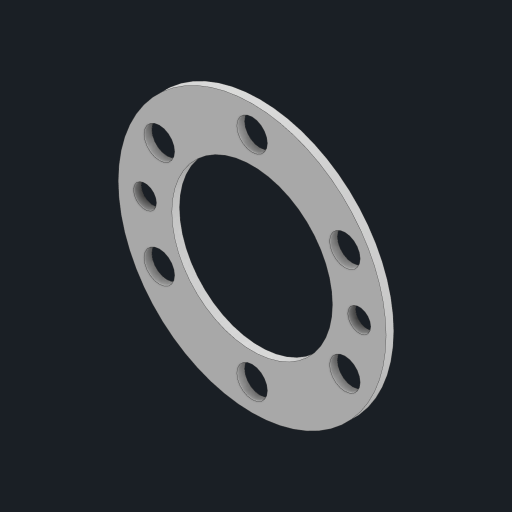
# Autodesk Inventor part: AK80Head
Saved by Autodesk Inventor 2023 (Build 270158000, 158)
## iProperties
Created: 2023-03-31
Part Number: AK80Head
Material: Generic
Document SubType Name: Modeling
Designer: valer
Density: 1 g/cm^3
Appearance: Default
Author: valer
Autodesk Inventor part; units mm, degrees
ref_plane "YZ Plane" through (0, 0, 0) normal (1, 0, 0) x (0, 1, 0)
ref_plane "XZ Plane" through (0, 0, 0) normal (0, 1, 0) x (-1, 0, 0)
sketch "Sketch1" plane through (0, 0, 0) normal (0, 0, 1) x (1, 0, 0)
  circle A0 centre (0, 0) radius 49
  circle A1 centre (0, 0) radius 44.5
  circle A2 centre (0, 0) radius 14 construction
  line L0 (0, 0) -> (0, 49.9271) construction
  line L1 (0, 0) -> (49, 0) construction
  line L2 (0, 0) -> (-49, 0) construction
  circle A3 centre (14, 0) radius 1.5
  circle A4 centre (-14, 0) radius 1.5
  circle A5 centre (0, 14) radius 2
  circle A6 centre (0, 44.5) radius 1.5
  circle A7 centre (44.5, 0) radius 1.5
  circle A8 centre (-44.5, 0) radius 1.5
  line L3 (0, 0) -> (-12.1244, 7) construction
  circle A9 centre (-12.1244, 7) radius 2
  circle A10 centre (12.1244, 7) radius 2
  circle A11 centre (0, -14) radius 2
  circle A12 centre (-12.1244, -7) radius 2
  circle A13 centre (12.1244, -7) radius 2
  line L4 (0, 0) -> (-31.4663, 31.4663) construction
  circle A14 centre (-31.4663, 31.4663) radius 1.5
  circle A15 centre (31.4663, 31.4663) radius 1.5
  circle A16 centre (0, -44.5) radius 1.5
  circle A17 centre (-31.4663, -31.4663) radius 1.5
  circle A18 centre (31.4663, -31.4663) radius 1.5
  circle A19 centre (0, 0) radius 10.5
  circle A20 centre (0, 0) radius 17.5
  circle A21 centre (0, 0) radius 36
  circle A22 centre (0, 0) radius 40
  circle A23 centre (0, 0) radius 5
  dimension "d0" = 98
  dimension "d1" = 89
  dimension "d2" = 28
  dimension "d3" = 3
  dimension "d4" = 3
  dimension "d5" = 4
  dimension "d6" = 3
  dimension "d7" = 3
  dimension "d8" = 3
  dimension "d9" = 30
  dimension "d10" = 60
  dimension "d11" = 4
  dimension "d12" = 45
  dimension "d13" = 3
  dimension "d14" = 21
  dimension "d15" = 35
  dimension "d16" = 72
  dimension "d17" = 80
  dimension "d18" = 10
  constraints: 24 centre point, 10 coincident, 10 end point, 10 point on circle, 8 symmetric about line, 6 point on line, 2 horizontal, 1 vertical, 8 other
  measures "d0" diameter of A0
  measures "d1" diameter of A1
  measures "d2" diameter of A2
  measures "d3" diameter of A3
  measures "d4" diameter of A4
  measures "d5" diameter of A5
  measures "d6" diameter of A6
  measures "d7" diameter of A7
  measures "d8" diameter of A8
  measures "d9" angle of L3 L2
  measures "d10" angle of L0 L3
  measures "d11" diameter of A9
  measures "d12" angle of L2 L4
  measures "d13" diameter of A14
  measures "d14" diameter of A19
  measures "d15" diameter of A20
  measures "d16" diameter of A21
  measures "d17" diameter of A22
  measures "d18" diameter of A23
extrude "Extrusion1" add sketch "Sketch1" along normal blind 1 contours A20
ref_plane "Work Plane1" through (0, 0, -8) normal (0, 0, 1) x (1, 0, 0)
sketch "Sketch2" plane through (0, 0, -8) normal (0, 0, 1) x (1, 0, 0)
  circle A0 centre (0, 0) radius 40 projected
loft "Loft1" add profiles "Sketch1", "Sketch2" contours A3 | A4 | A5 | A9 | A10 | A11 | A12 | A13 | A19 | A20 | A21 | A23 / all
sketch "Sketch3" plane through (0, 0, -8) normal (0, 0, 1) x (1, 0, 0)
  circle A0 centre (0, 0) radius 49 projected
extrude "Extrusion2" add sketch "Sketch3" against normal blind 42.7
hole "Hole1" at (-44.5, 0, 0) at (-31.4663, 31.4663, 0) at (0, 44.5, 0) at (31.4663, 31.4663, 0) at (44.5, 0, 0) at (31.4663, -31.4663, 0) at (0, -44.5, 0) at (-31.4663, -31.4663, 0) direction (0, 0, -1) diameter 3 depth 8 tip angle 118
move faces "Move1" translate (0, 0, -8) faces at (1.689, -2.0915, 0)
sketch "Sketch4" plane through (0, 0, -50.7) normal (0, 0, -1) x (-1, 0, 0)
  line L0 (0, 0) -> (-47.3304, -12.6821) construction
  circle A0 centre (0, 0) radius 49 projected
  line L1 (0, 0) -> (12.6821, -47.3304) construction
  circle A1 centre (0, 0) radius 49 projected
  line L2 (0, 0) -> (-12.6821, 47.3304) construction
  circle A2 centre (0, 0) radius 42.5 construction
  circle A3 centre (10.9998, -41.0518) radius 1.5
  circle A4 centre (0, 0) radius 17.5 construction
  line L3 (0, 0) -> (-24.5, -42.4352) construction
  circle A5 centre (-21.25, -36.8061) radius 1.5
  circle A6 centre (-41.0518, -10.9998) radius 1.5
  circle A7 centre (-36.8061, 21.25) radius 1.5
  circle A8 centre (-10.9998, 41.0518) radius 1.5
  circle A9 centre (36.8061, -21.25) radius 1.5
  circle A10 centre (41.0518, 10.9998) radius 1.5
  circle A11 centre (21.25, 36.8061) radius 1.5
  line L4 (0, -68.6) -> (0, 68.6) construction
  dimension "d38" = 85
  dimension "d40" = 3
  dimension "d41" = 45
  dimension "d53" = 15
  constraints: 9 centre point, 8 end point, 6 point on circle, 5 symmetric about line, 3 point on line, 2 equal radius, 2 perpendicular, 1 coincident, 7 other
  measures "d38" diameter of A2
  measures "d40" diameter of A3
  measures "d41" angle of L3 L1
  measures "d53" angle of L4 L2
hole "Hole2" at (-10.9998, -41.0518, -50.7) at (-36.8061, -21.25, -50.7) at (21.25, -36.8061, -50.7) at (41.0518, -10.9998, -50.7) at (-41.0518, 10.9998, -50.7) at (-21.25, 36.8061, -50.7) at (10.9998, 41.0518, -50.7) at (36.8061, 21.25, -50.7) direction (0, 0, 1) diameter 3 depth 8 tip angle 118
sketch "Sketch5" plane through (0, 0, -50.7) normal (0, 0, -1) x (-1, 0, 0)
  circle A0 centre (0, 0) radius 35.32
  dimension "d49" = 70.64
  constraints: 1 centre point, 1 coincident
  measures "d49" diameter of A0
extrude "Extrusion3" add sketch "Sketch5" along normal blind 11.2
split "Sculpt1" plane through (0, 0, 0) removes the side toward (0, 0, -1)
body "Solid1"
